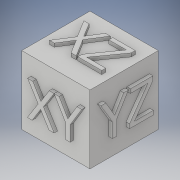
# Autodesk Inventor part: test_cube
Saved by Autodesk Inventor 2018 (Build 220112000, 112)
## iProperties
Created: 2017-11-05
Part Number: test_cube
Material: Generisch
Document SubType Name: Blech
Designer: t.pietrowski
Density: 1 g/cm^3
Sheet Metal Rule: Standard_mm
Appearance: Vorgabe
Author: t.pietrowski
Autodesk Inventor part; units mm, degrees
ref_plane "YZ Plane" through (0, 0, 0) normal (1, 0, 0) x (0, 1, 0)
ref_plane "XZ Plane" through (0, 0, 0) normal (0, 1, 0) x (-1, 0, 0)
ref_plane "XY Plane" through (0, 0, 0) normal (0, 0, 1) x (1, 0, 0)
sketch "Skizze1" plane through (0, 0, 0) normal (0, 1, 0) x (-1, 0, 0)
  line L0 (9.5031, 9.441) -> (-10.4969, 9.441)
  line L1 (-10.4969, 9.441) -> (-10.4969, -10.559)
  line L2 (-10.4969, -10.559) -> (9.5031, -10.559)
  line L3 (9.5031, -10.559) -> (9.5031, 9.441)
  point P0 (0, 0)
  dimension "d0" = 20
  dimension "d1" = 20
  constraints: 8 end point, 2 parallel, 1 horizontal, 1 perpendicular
  measures "d0" distance of L0.end L1.end
  measures "d1" distance of L1.end L2.end
extrude "Extrusion1" add sketch "Skizze1" along normal mid plane 20
sketch "Skizze2" plane through (0, -10, 0) normal (0, -1, 0) x (1, 0, 0)
  line L0 (-6.9201, 4.3012) -> (5.6278, 4.3012) construction
  line L1 (5.6278, 4.3012) -> (5.6278, -4.2448) construction
  line L2 (5.6278, -4.2448) -> (-6.9201, -4.2448) construction
  line L3 (-6.9201, -4.2448) -> (-6.9201, 4.3012) construction
  line L4 (1.0053, -5.6988) -> (-0.5182, -5.6988)
  line L5 (-0.5182, -5.6988) -> (-2.9493, -1.7118)
  line L6 (-2.9493, -1.7118) -> (-5.4291, -5.6988)
  line L7 (-5.4291, -5.6988) -> (-6.8634, -5.6988)
  line L8 (-6.8634, -5.6988) -> (-3.6786, -0.6907)
  line L9 (-3.6786, -0.6907) -> (-6.7662, 4.3012)
  line L10 (-6.7662, 4.3012) -> (-5.2427, 4.3012)
  line L11 (-5.2427, 4.3012) -> (-2.8602, 0.3871)
  line L12 (-2.8602, 0.3871) -> (-0.4291, 4.3012)
  line L13 (-0.4291, 4.3012) -> (1.0053, 4.3012)
  line L14 (1.0053, 4.3012) -> (-2.1227, -0.6259)
  line L15 (-2.1227, -0.6259) -> (1.0053, -5.6988)
  line L16 (9.0766, 4.3012) -> (5.6974, -1.2742)
  line L17 (5.6974, -1.2742) -> (5.6974, -5.6988)
  line L18 (5.6974, -5.6988) -> (4.3684, -5.6988)
  line L19 (4.3684, -5.6988) -> (4.3684, -1.412)
  line L20 (4.3684, -1.412) -> (0.9891, 4.3012)
  line L21 (0.9891, 4.3012) -> (2.464, 4.3012)
  line L22 (2.464, 4.3012) -> (5.041, -0.0992)
  line L23 (5.041, -0.0992) -> (7.6666, 4.3012)
  line L24 (7.6666, 4.3012) -> (9.0766, 4.3012)
  point P0 (0, 0)
  constraints: 2 other
emboss "Prägen1" sketch "Skizze2" operation add depth 1 direction (0, 1, 0)
sketch "Skizze3" plane through (-9.5031, 10, 9.441) normal (0, 0, 1) x (1, 0, 0)
  line L0 (2.4004, -4.3596) -> (17.6852, -4.3596) construction
  line L1 (17.6852, -4.3596) -> (17.6852, -18.9828) construction
  line L2 (17.6852, -18.9828) -> (2.4004, -18.9828) construction
  line L3 (2.4004, -18.9828) -> (2.4004, -4.3596) construction
  line L4 (10.3258, -14.3596) -> (8.8023, -14.3596)
  line L5 (8.8023, -14.3596) -> (6.3712, -10.3726)
  line L6 (6.3712, -10.3726) -> (3.8915, -14.3596)
  line L7 (3.8915, -14.3596) -> (2.4571, -14.3596)
  line L8 (2.4571, -14.3596) -> (5.6419, -9.3515)
  line L9 (5.6419, -9.3515) -> (2.5544, -4.3596)
  line L10 (2.5544, -4.3596) -> (4.0779, -4.3596)
  line L11 (4.0779, -4.3596) -> (6.4604, -8.2737)
  line L12 (6.4604, -8.2737) -> (8.8915, -4.3596)
  line L13 (8.8915, -4.3596) -> (10.3258, -4.3596)
  line L14 (10.3258, -4.3596) -> (7.1978, -9.2867)
  line L15 (7.1978, -9.2867) -> (10.3258, -14.3596)
  line L16 (17.7732, -14.3596) -> (10.7878, -14.3596)
  line L17 (10.7878, -14.3596) -> (10.7878, -13.1197)
  line L18 (10.7878, -13.1197) -> (16.1362, -5.5428)
  line L19 (16.1362, -5.5428) -> (11.0309, -5.5428)
  line L20 (11.0309, -5.5428) -> (11.0309, -4.3596)
  line L21 (11.0309, -4.3596) -> (17.6354, -4.3596)
  line L22 (17.6354, -4.3596) -> (17.6354, -5.559)
  line L23 (17.6354, -5.559) -> (12.2302, -13.1765)
  line L24 (12.2302, -13.1765) -> (17.7732, -13.1765)
  line L25 (17.7732, -13.1765) -> (17.7732, -14.3596)
  point P0 (9.5031, -10)
  constraints: 2 other
emboss "Prägen2" sketch "Skizze3" operation add depth 1 direction (0, 0, -1)
sketch "Skizze4" plane through (10.4969, -10, -10.559) normal (1, 0, 0) x (0, 0, -1)
  line L0 (-15.3986, 2.2358) -> (-15.3986, 16.7197) construction
  line L1 (-15.3986, 16.7197) -> (-0.1138, 16.7197) construction
  line L2 (-0.1138, 16.7197) -> (-0.1138, 2.2358) construction
  line L3 (-0.1138, 2.2358) -> (-15.3986, 2.2358) construction
  line L4 (-15.3986, 10.2503) -> (-9.8232, 6.8711)
  line L5 (-9.8232, 6.8711) -> (-5.3986, 6.8711)
  line L6 (-5.3986, 6.8711) -> (-5.3986, 5.5421)
  line L7 (-5.3986, 5.5421) -> (-9.6855, 5.5421)
  line L8 (-9.6855, 5.5421) -> (-15.3986, 2.1628)
  line L9 (-15.3986, 2.1628) -> (-15.3986, 3.6377)
  line L10 (-15.3986, 3.6377) -> (-10.9983, 6.2147)
  line L11 (-10.9983, 6.2147) -> (-15.3986, 8.8403)
  line L12 (-15.3986, 8.8403) -> (-15.3986, 10.2503)
  line L13 (-5.3986, 17.5518) -> (-5.3986, 10.5664)
  line L14 (-5.3986, 10.5664) -> (-6.6385, 10.5664)
  line L15 (-6.6385, 10.5664) -> (-14.2155, 15.9149)
  line L16 (-14.2155, 15.9149) -> (-14.2155, 10.8095)
  line L17 (-14.2155, 10.8095) -> (-15.3986, 10.8095)
  line L18 (-15.3986, 10.8095) -> (-15.3986, 17.414)
  line L19 (-15.3986, 17.414) -> (-14.1992, 17.414)
  line L20 (-14.1992, 17.414) -> (-6.5817, 12.0089)
  line L21 (-6.5817, 12.0089) -> (-6.5817, 17.5518)
  line L22 (-6.5817, 17.5518) -> (-5.3986, 17.5518)
  point P0 (-10.559, 10)
  constraints: 2 other
emboss "Prägen3" sketch "Skizze4" operation add depth 1 direction (-1, 0, 0)
equation "\"Biegeradius\" = Stärke"
equation "\"BreiteBiegungsfreistellung\" = Stärke"
equation "\"TiefeBiegungsfreistellung\" = 0.5 * Stärke"
equation "\"GrößeEckenfreistellung\" = 4 * Stärke"
equation "\"MinimalRest\" = 2 * Stärke"
equation "\"Übergangsradius\" = Biegeradius"
equation "\"JacobiRadiusGröße\" = Biegeradius"
equation "\"Abstandsgröße\" = Stärke"
equation "\"Stärke\" = 0.5"
